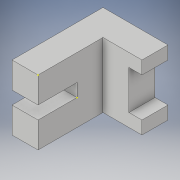
# Autodesk Inventor part: Model Creation 3
Saved by Autodesk Inventor 2019 (Build 230136000, 136)
## iProperties
Created: 2019-09-09
Part Number: Model Creation 3
Material: Generic
Document SubType Name: Modeling
Designer: IED8
Density: 1 g/cm^3
Appearance: Default
Author: IED8
Autodesk Inventor part; units mm, degrees
ref_plane "YZ Plane" through (0, 0, 0) normal (1, 0, 0) x (0, 1, 0)
ref_plane "XZ Plane" through (0, 0, 0) normal (0, 1, 0) x (-1, 0, 0)
ref_plane "XY Plane" through (0, 0, 0) normal (0, 0, 1) x (1, 0, 0)
sketch "Sketch1" plane through (0, 0, 0) normal (1, 0, 0) x (0, 1, 0)
  line L0 (0, 0) -> (0, -88.9)
  line L1 (0, -88.9) -> (-63.5, -88.9)
  line L2 (-63.5, -88.9) -> (-63.5, 0)
  line L3 (-63.5, 0) -> (0, 0)
  dimension "d0" = 88.9
  dimension "d1" = 63.5
  constraints: 8 end point, 3 perpendicular, 1 vertical
  measures "d0" distance of L0.start L0.end
  measures "d1" distance of L0.end L1.end
extrude "Extrusion1" add sketch "Sketch1" along normal blind 25.4
sketch "Sketch2" plane through (25.4, 0, 0) normal (1, 0, 0) x (0, 0, -1)
  point P0 (0, 0)
sketch "Sketch3" plane through (25.4, 0, 0) normal (1, 0, 0) x (0, 0, -1)
  line L0 (0, 0) -> (0, -63.5) projected
  line L1 (0, -25.4) -> (38.1, -25.4)
  line L2 (38.1, -25.4) -> (38.1, -38.1)
  line L3 (38.1, -38.1) -> (0, -38.1)
  line L4 (0, -25.4) -> (0, -38.1)
  dimension "d4" = 25.4
  dimension "d5" = 38.1
  dimension "d6" = 12.7
  constraints: 8 end point, 2 perpendicular, 2 point on line, 1 collinear
  measures "d4" distance of L0.start L1.start
  measures "d5" distance of L1.start L1.end
  measures "d6" distance of L1.end L2.end
extrude "Extrusion2" cut sketch "Sketch3" against normal blind 25.4
sketch "Sketch4" plane through (25.4, 0, 0) normal (1, 0, 0) x (0, 0, -1)
  line L0 (0, 0) -> (88.9, 0) projected
  line L1 (88.9, 0) -> (63.5, 0)
  line L2 (63.5, 0) -> (63.5, -63.5)
  line L3 (0, -63.5) -> (88.9, -63.5) projected
  line L4 (63.5, -63.5) -> (88.9, -63.5)
  line L5 (88.9, -63.5) -> (88.9, 0)
  dimension "d9" = 25.4
  constraints: 8 end point, 2 perpendicular, 2 point on line, 1 collinear
  measures "d9" distance of L0.end L1.end
extrude "Extrusion3" add sketch "Sketch4" along normal blind 38.1
sketch "Sketch5" plane through (63.5, 0, 0) normal (1, 0, 0) x (0, 0, -1)
  point P0 (0, 0)
sketch "Sketch6" plane through (63.5, 0, 0) normal (1, 0, 0) x (0, 0, -1)
  line L0 (63.5, -12.7) -> (88.9, -12.7)
  line L1 (88.9, -12.7) -> (88.9, -50.8)
  line L2 (88.9, -63.5) -> (88.9, 0) projected
  line L3 (88.9, -50.8) -> (63.5, -50.8)
  line L4 (63.5, -63.5) -> (63.5, 0) projected
  line L5 (63.5, -12.7) -> (63.5, -50.8)
  point P0 (0, 0)
  dimension "d12" = 12.7
  dimension "d13" = 38.1
  constraints: 8 end point, 2 perpendicular, 2 point on line
  measures "d12" distance of L4.end L0.start
  measures "d13" distance of L0.end L1.end
extrude "Extrusion4" cut sketch "Sketch6" against normal blind 12.7
body "Solid1"
